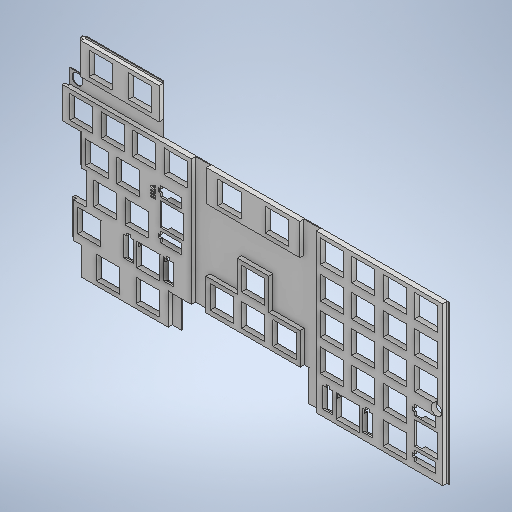
# Autodesk Inventor part: Right Plate
Saved by Autodesk Inventor 2025 (Build 290162000, 162)
## iProperties
Created: 2024-08-20
Part Number: Right Plate
Material: Generic
Document SubType Name: Modeling
Designer: adam
Density: 1 g/cm^3
Appearance: Default
Author: adam
Autodesk Inventor part; units mm, degrees
(part 1 of 2)
ref_plane "YZ Plane" through (0, 0, 0) normal (1, 0, 0) x (0, 1, 0)
ref_plane "XZ Plane" through (0, 0, 0) normal (0, 1, 0) x (-1, 0, 0)
ref_plane "XY Plane" through (0, 0, 0) normal (0, 0, 1) x (1, 0, 0)
sketch "Sketch1" plane through (0, 0, 0) normal (0, 0, 1) x (1, 0, 0)
  line L0 (490, -165) -> (40, -165) projected
  line L1 (490, -40) -> (490, -165) projected
  line L2 (40, -40) -> (490, -40) projected
  line L3 (40, -165) -> (40, -40) projected
  circle A0 centre (62.4608, -160.0704) radius 0.725 projected
  circle A1 centre (69.4608, -161.1204) radius 0.725 projected
  circle A2 centre (66.8608, -155.3704) radius 2.55 projected
  circle A3 centre (86.3368, -160.0704) radius 0.725 projected
  circle A4 centre (93.3368, -161.1204) radius 0.725 projected
  circle A5 centre (90.7368, -155.3704) radius 2.55 projected
  line L4 (118.6501, -160.3704) -> (124.6501, -160.3704) projected
  line L5 (118.6501, -145.3704) -> (118.6501, -160.3704) projected
  line L6 (124.6501, -145.3704) -> (118.6501, -145.3704) projected
  line L7 (124.6501, -160.3704) -> (124.6501, -145.3704) projected
  circle A6 centre (53.5708, -141.0204) radius 0.725 projected
  circle A7 centre (60.5708, -142.0704) radius 0.725 projected
  circle A8 centre (79.7328, -141.0204) radius 0.725 projected
  circle A9 centre (86.7328, -142.0704) radius 0.725 projected
  circle A10 centre (57.9708, -136.3204) radius 2.55 projected
  circle A11 centre (84.1328, -136.3204) radius 2.55 projected
  circle A12 centre (105.7828, -142.0704) radius 0.725 projected
  circle A13 centre (98.7828, -141.0204) radius 0.725 projected
  circle A14 centre (124.8328, -142.0704) radius 0.725 projected
  circle A15 centre (117.8328, -141.0204) radius 0.725 projected
  circle A16 centre (136.8828, -141.0204) radius 0.725 projected
  circle A17 centre (143.8828, -142.0704) radius 0.725 projected
  circle A18 centre (103.1828, -136.3204) radius 2.55 projected
  circle A19 centre (122.2328, -136.3204) radius 2.55 projected
  circle A20 centre (141.2828, -136.3204) radius 2.55 projected
  circle A21 centre (155, -160) radius 1.75 projected
  circle A22 centre (184.0001, -160.0704) radius 0.725 projected
  circle A23 centre (191.0001, -161.1204) radius 0.725 projected
  circle A24 centre (188.4001, -155.3704) radius 2.55 projected
  line L8 (252.1501, -160.3704) -> (258.1501, -160.3704) projected
  line L9 (252.1501, -145.3704) -> (252.1501, -160.3704) projected
  line L10 (258.1501, -145.3704) -> (252.1501, -145.3704) projected
  line L11 (258.1501, -160.3704) -> (258.1501, -145.3704) projected
  circle A25 centre (162.9328, -142.0704) radius 0.725 projected
  circle A26 centre (155.9328, -141.0204) radius 0.725 projected
  circle A27 centre (174.9828, -141.0204) radius 0.725 projected
  circle A28 centre (181.9828, -142.0704) radius 0.725 projected
  circle A29 centre (194.0328, -141.0204) radius 0.725 projected
  circle A30 centre (201.0328, -142.0704) radius 0.725 projected
  circle A31 centre (160.3328, -136.3204) radius 2.55 projected
  circle A32 centre (179.3828, -136.3204) radius 2.55 projected
  circle A33 centre (198.4328, -136.3204) radius 2.55 projected
  circle A34 centre (220.0828, -142.0704) radius 0.725 projected
  circle A35 centre (213.0828, -141.0204) radius 0.725 projected
  circle A36 centre (232.1368, -141.0224) radius 0.725 projected
  circle A37 centre (239.1368, -142.0724) radius 0.725 projected
  circle A38 centre (258.1768, -142.0924) radius 0.725 projected
  circle A39 centre (251.1768, -141.0424) radius 0.725 projected
  circle A40 centre (217.4828, -136.3204) radius 2.55 projected
  circle A41 centre (236.5368, -136.3224) radius 2.55 projected
  circle A42 centre (255.5768, -136.3424) radius 2.55 projected
  circle A43 centre (45, -127) radius 1.75 projected
  circle A44 centre (55.7448, -123.0204) radius 0.725 projected
  circle A45 centre (48.7448, -121.9704) radius 0.725 projected
  circle A46 centre (70.0808, -121.9704) radius 0.725 projected
  circle A47 centre (53.1448, -117.2704) radius 2.55 projected
  circle A48 centre (77.0808, -123.0204) radius 0.725 projected
  circle A49 centre (96.1308, -123.0204) radius 0.725 projected
  circle A50 centre (89.1308, -121.9704) radius 0.725 projected
  circle A51 centre (74.4808, -117.2704) radius 2.55 projected
  circle A52 centre (93.5308, -117.2704) radius 2.55 projected
  circle A53 centre (108.1808, -121.9704) radius 0.725 projected
  circle A54 centre (115.1808, -123.0204) radius 0.725 projected
  circle A55 centre (112.5808, -117.2704) radius 2.55 projected
  circle A56 centre (134.2308, -123.0204) radius 0.725 projected
  circle A57 centre (127.2308, -121.9704) radius 0.725 projected
  circle A58 centre (153.2808, -123.0204) radius 0.725 projected
  circle A59 centre (146.2808, -121.9704) radius 0.725 projected
  circle A60 centre (131.6308, -117.2704) radius 2.55 projected
  circle A61 centre (150.6808, -117.2704) radius 2.55 projected
  circle A62 centre (55.8568, -102.9204) radius 0.725 projected
  circle A63 centre (62.8568, -103.9704) radius 0.725 projected
  circle A64 centre (84.3048, -102.9204) radius 0.725 projected
  circle A65 centre (91.3048, -103.9704) radius 0.725 projected
  circle A66 centre (103.3548, -102.9204) radius 0.725 projected
  circle A67 centre (110.3548, -103.9704) radius 0.725 projected
  circle A68 centre (122.4048, -102.9204) radius 0.725 projected
  circle A69 centre (129.4048, -103.9704) radius 0.725 projected
  circle A70 centre (141.4548, -102.9204) radius 0.725 projected
  circle A71 centre (148.4548, -103.9704) radius 0.725 projected
  circle A72 centre (165.3308, -121.9704) radius 0.725 projected
  circle A73 centre (172.3308, -123.0204) radius 0.725 projected
  circle A74 centre (169.7308, -117.2704) radius 2.55 projected
  circle A75 centre (191.3808, -123.0204) radius 0.725 projected
  circle A76 centre (184.3808, -121.9704) radius 0.725 projected
  circle A77 centre (203.4308, -121.9704) radius 0.725 projected
  circle A78 centre (188.7808, -117.2704) radius 2.55 projected
  circle A79 centre (207.8308, -117.2704) radius 2.55 projected
  circle A80 centre (210.4308, -123.0204) radius 0.725 projected
  circle A81 centre (222.4808, -121.9704) radius 0.725 projected
  circle A82 centre (229.4808, -123.0204) radius 0.725 projected
  circle A83 centre (226.8808, -117.2704) radius 2.55 projected
  circle A84 centre (248.5308, -123.0204) radius 0.725 projected
  circle A85 centre (241.5308, -121.9704) radius 0.725 projected
  circle A86 centre (260.8348, -121.9704) radius 0.725 projected
  circle A87 centre (245.9308, -117.2704) radius 2.55 projected
  circle A88 centre (167.5048, -104.0492) radius 0.725 projected
  circle A89 centre (160.5048, -102.9992) radius 0.725 projected
  circle A90 centre (179.5548, -102.9204) radius 0.725 projected
  circle A91 centre (186.5548, -103.9704) radius 0.725 projected
  circle A92 centre (198.6048, -102.9204) radius 0.725 projected
  circle A93 centre (205.6048, -103.9704) radius 0.725 projected
  circle A94 centre (217.6548, -102.9204) radius 0.725 projected
  circle A95 centre (224.6548, -103.9704) radius 0.725 projected
  circle A96 centre (236.7048, -102.9204) radius 0.725 projected
  circle A97 centre (243.7048, -103.9704) radius 0.725 projected
  circle A98 centre (255.7548, -102.9204) radius 0.725 projected
  circle A99 centre (262.7548, -103.9704) radius 0.725 projected
  circle A100 centre (265, -160) radius 1.75 projected
  circle A101 centre (281.6628, -160.0704) radius 0.725 projected
  circle A102 centre (288.6628, -161.1204) radius 0.725 projected
  circle A103 centre (286.0628, -155.3704) radius 2.55 projected
  circle A104 centre (305.5388, -160.0704) radius 0.725 projected
  circle A105 centre (312.5388, -161.1204) radius 0.725 projected
  circle A106 centre (309.9388, -155.3704) radius 2.55 projected
  circle A107 centre (375, -160) radius 1.75 projected
  circle A108 centre (277.2328, -142.0704) radius 0.725 projected
  circle A109 centre (270.2328, -141.0204) radius 0.725 projected
  circle A110 centre (306.0468, -141.0204) radius 0.725 projected
  circle A111 centre (313.0468, -142.0704) radius 0.725 projected
  circle A112 centre (274.6328, -136.3204) radius 2.55 projected
  circle A113 centre (310.4468, -136.3204) radius 2.55 projected
  line L12 (295.4468, -141.3204) -> (301.4468, -141.3204) projected
  line L13 (295.4468, -126.3204) -> (295.4468, -141.3204) projected
  line L14 (301.4468, -126.3204) -> (295.4468, -126.3204) projected
  line L15 (301.4468, -141.3204) -> (301.4468, -126.3204) projected
  circle A114 centre (357.43, -142.0196) radius 0.725 projected
  circle A115 centre (350.43, -140.9696) radius 0.725 projected
  circle A116 centre (369.48, -140.9696) radius 0.725 projected
  line L16 (319.4468, -141.3204) -> (325.4468, -141.3204) projected
  line L17 (319.4468, -126.3204) -> (319.4468, -141.3204) projected
  line L18 (325.4468, -126.3204) -> (319.4468, -126.3204) projected
  line L19 (325.4468, -141.3204) -> (325.4468, -126.3204) projected
  circle A117 centre (354.83, -136.2696) radius 2.55 projected
  circle A118 centre (373.88, -136.2696) radius 2.55 projected
  circle A119 centre (426.8108, -160.0704) radius 0.725 projected
  circle A120 centre (431.2108, -155.3704) radius 2.55 projected
  line L20 (416.2108, -160.3704) -> (422.2108, -160.3704) projected
  line L21 (416.2108, -145.3704) -> (416.2108, -160.3704) projected
  line L22 (422.2108, -145.3704) -> (416.2108, -145.3704) projected
  line L23 (422.2108, -160.3704) -> (422.2108, -145.3704) projected
  circle A121 centre (433.8108, -161.1204) radius 0.725 projected
  circle A122 centre (455.2588, -160.0704) radius 0.725 projected
  circle A123 centre (462.2588, -161.1204) radius 0.725 projected
  circle A124 centre (459.6588, -155.3704) radius 2.55 projected
  line L24 (468.7088, -160.774) -> (483.7088, -160.774) projected
  line L25 (468.7088, -154.774) -> (468.7088, -160.774) projected
  line L26 (483.7088, -154.774) -> (468.7088, -154.774) projected
  line L27 (483.7088, -160.774) -> (483.7088, -154.774) projected
  line L28 (440.2108, -160.3704) -> (446.2108, -160.3704) projected
  line L29 (440.2108, -145.3704) -> (440.2108, -160.3704) projected
  line L30 (446.2108, -145.3704) -> (440.2108, -145.3704) projected
  line L31 (446.2108, -160.3704) -> (446.2108, -145.3704) projected
  circle A125 centre (483.4088, -150.174) radius 0.725 projected
  circle A126 centre (376.48, -142.0196) radius 0.725 projected
  circle A127 centre (388.53, -140.9696) radius 0.725 projected
  circle A128 centre (395.53, -142.0196) radius 0.725 projected
  circle A129 centre (417.1588, -140.922) radius 0.725 projected
  circle A130 centre (424.1588, -141.972) radius 0.725 projected
  circle A131 centre (392.93, -136.2696) radius 2.55 projected
  circle A132 centre (421.5588, -136.222) radius 2.55 projected
  circle A133 centre (443.2088, -141.972) radius 0.725 projected
  circle A134 centre (436.2088, -140.922) radius 0.725 projected
  circle A135 centre (455.2588, -140.922) radius 0.725 projected
  circle A136 centre (478.7088, -145.774) radius 2.55 projected
  circle A137 centre (462.2588, -141.972) radius 0.725 projected
  circle A138 centre (484.4588, -143.174) radius 0.725 projected
  circle A139 centre (440.6088, -136.222) radius 2.55 projected
  circle A140 centre (459.6588, -136.222) radius 2.55 projected
  line L32 (468.7088, -136.774) -> (483.7088, -136.774) projected
  line L33 (468.7088, -130.774) -> (468.7088, -136.774) projected
  line L34 (483.7088, -130.774) -> (468.7088, -130.774) projected
  line L35 (483.7088, -136.774) -> (483.7088, -130.774) projected
  circle A141 centre (267.8348, -123.0204) radius 0.725 projected
  circle A142 centre (286.8848, -123.0204) radius 0.725 projected
  circle A143 centre (279.8848, -121.9704) radius 0.725 projected
  circle A144 centre (265.2348, -117.2704) radius 2.55 projected
  circle A145 centre (284.2848, -117.2704) radius 2.55 projected
  circle A146 centre (305.9348, -123.0204) radius 0.725 projected
  circle A147 centre (298.9348, -121.9704) radius 0.725 projected
  circle A148 centre (303.3348, -117.2704) radius 2.55 projected
  line L36 (315.6708, -122.8724) -> (330.3933, -122.8724)
  line L37 (315.6708, -116.8724) -> (315.6708, -122.8724) projected
  line L38 (330.3933, -116.8724) -> (315.6708, -116.8724)
  line L39 (330.3933, -122.8724) -> (330.3933, -116.8724)
  circle A149 centre (369.48, -121.9196) radius 0.725 projected
  circle A150 centre (373.88, -117.2196) radius 2.55 projected
  circle A151 centre (274.8048, -102.9204) radius 0.725 projected
  circle A152 centre (281.8048, -103.9704) radius 0.725 projected
  circle A153 centre (293.8548, -102.9204) radius 0.725 projected
  circle A154 centre (300.8548, -103.9704) radius 0.725 projected
  circle A155 centre (329.3458, -112.2974) radius 0.725 projected
  circle A156 centre (324.6458, -107.8974) radius 2.55 projected
  circle A157 centre (330.3958, -105.2974) radius 0.725 projected
  circle A158 centre (376.48, -122.9696) radius 0.725 projected
  circle A159 centre (417.1588, -121.872) radius 0.725 projected
  circle A160 centre (424.1588, -122.922) radius 0.725 projected
  circle A161 centre (421.5588, -117.172) radius 2.55 projected
  circle A162 centre (485, -127) radius 1.75 projected
  circle A163 centre (443.2088, -122.922) radius 0.725 projected
  circle A164 centre (436.2088, -121.872) radius 0.725 projected
  circle A165 centre (455.2588, -121.872) radius 0.725 projected
  circle A166 centre (440.6088, -117.172) radius 2.55 projected
  circle A167 centre (462.2588, -122.922) radius 0.725 projected
  circle A168 centre (481.3088, -122.922) radius 0.725 projected
  circle A169 centre (474.3088, -121.872) radius 0.725 projected
  circle A170 centre (459.6588, -117.172) radius 2.55 projected
  circle A171 centre (478.7088, -117.172) radius 2.55 projected
  circle A172 centre (417.1588, -102.822) radius 0.725 projected
  circle A173 centre (424.1588, -103.872) radius 0.725 projected
  circle A174 centre (436.2088, -102.822) radius 0.725 projected
  circle A175 centre (443.2088, -103.872) radius 0.725 projected
  circle A176 centre (455.2588, -102.822) radius 0.725 projected
  circle A177 centre (462.2588, -103.872) radius 0.725 projected
  circle A178 centre (474.3088, -102.822) radius 0.725 projected
  circle A179 centre (481.3088, -103.872) radius 0.725 projected
  line L40 (45.2568, -103.2204) -> (51.2568, -103.2204) projected
  line L41 (45.2568, -88.2204) -> (45.2568, -103.2204) projected
  line L42 (51.2568, -88.2204) -> (45.2568, -88.2204) projected
  line L43 (51.2568, -103.2204) -> (51.2568, -88.2204) projected
  circle A180 centre (60.2568, -98.2204) radius 2.55 projected
  line L44 (69.2568, -103.2204) -> (75.2568, -103.2204) projected
  line L45 (69.2568, -88.2204) -> (69.2568, -103.2204) projected
  line L46 (75.2568, -88.2204) -> (69.2568, -88.2204) projected
  line L47 (75.2568, -103.2204) -> (75.2568, -88.2204) projected
  circle A181 centre (88.7048, -98.2204) radius 2.55 projected
  circle A182 centre (107.7548, -98.2204) radius 2.55 projected
  circle A183 centre (126.8048, -98.2204) radius 2.55 projected
  circle A184 centre (145.8548, -98.2204) radius 2.55 projected
  circle A185 centre (51.1288, -83.8704) radius 0.725 projected
  circle A186 centre (58.1288, -84.9204) radius 0.725 projected
  circle A187 centre (74.9068, -83.8704) radius 0.725 projected
  circle A188 centre (81.9068, -84.9204) radius 0.725 projected
  circle A189 centre (93.9568, -83.8704) radius 0.725 projected
  circle A190 centre (55.5288, -79.1704) radius 2.55 projected
  circle A191 centre (79.3068, -79.1704) radius 2.55 projected
  circle A192 centre (98.3568, -79.1704) radius 2.55 projected
  circle A193 centre (100.9568, -84.9204) radius 0.725 projected
  circle A194 centre (113.0068, -83.8704) radius 0.725 projected
  circle A195 centre (120.0068, -84.9204) radius 0.725 projected
  circle A196 centre (132.0568, -83.8704) radius 0.725 projected
  circle A197 centre (139.0568, -84.9204) radius 0.725 projected
  circle A198 centre (151.1068, -83.8704) radius 0.725 projected
  circle A199 centre (117.4068, -79.1704) radius 2.55 projected
  circle A200 centre (136.4568, -79.1704) radius 2.55 projected
  circle A201 centre (164.9048, -98.2992) radius 2.55 projected
  circle A202 centre (183.9548, -98.2204) radius 2.55 projected
  circle A203 centre (203.0048, -98.2204) radius 2.55 projected
  circle A204 centre (222.0548, -98.2204) radius 2.55 projected
  circle A205 centre (241.1048, -98.2204) radius 2.55 projected
  circle A206 centre (260.1548, -98.2204) radius 2.55 projected
  circle A207 centre (158.1068, -84.9204) radius 0.725 projected
  circle A208 centre (170.1568, -83.8704) radius 0.725 projected
  circle A209 centre (177.1568, -84.9204) radius 0.725 projected
  circle A210 centre (189.2068, -83.8704) radius 0.725 projected
  circle A211 centre (196.2068, -84.9204) radius 0.725 projected
  circle A212 centre (208.2568, -83.8704) radius 0.725 projected
  circle A213 centre (155.5068, -79.1704) radius 2.55 projected
  circle A214 centre (174.5568, -79.1704) radius 2.55 projected
  circle A215 centre (193.6068, -79.1704) radius 2.55 projected
  circle A216 centre (215.2568, -84.9204) radius 0.725 projected
  circle A217 centre (227.3068, -83.8704) radius 0.725 projected
  circle A218 centre (234.3068, -84.9204) radius 0.725 projected
  circle A219 centre (246.3568, -83.8704) radius 0.725 projected
  circle A220 centre (253.3568, -84.9204) radius 0.725 projected
  circle A221 centre (212.6568, -79.1704) radius 2.55 projected
  circle A222 centre (231.7068, -79.1704) radius 2.55 projected
  circle A223 centre (250.7568, -79.1704) radius 2.55 projected
  circle A224 centre (45, -64.8616) radius 1.75 projected
  circle A225 centre (50.8588, -50.6116) radius 2.55 projected
  circle A226 centre (81.9072, -50.3984) radius 2.55 projected
  circle A227 centre (48.2588, -44.8616) radius 0.725 projected
  circle A228 centre (55.2588, -45.9116) radius 0.725 projected
  circle A229 centre (79.3072, -44.6484) radius 0.725 projected
  circle A230 centre (86.3072, -45.6984) radius 0.725 projected
  circle A231 centre (105.7228, -50.5136) radius 2.55 projected
  circle A232 centre (129.5988, -50.5416) radius 2.55 projected
  circle A233 centre (153.4748, -50.5136) radius 2.55 projected
  circle A234 centre (103.1228, -44.7636) radius 0.725 projected
  circle A235 centre (110.1228, -45.8136) radius 0.725 projected
  circle A236 centre (126.9988, -44.7916) radius 0.725 projected
  circle A237 centre (133.9988, -45.8416) radius 0.725 projected
  circle A238 centre (150.8748, -44.7636) radius 0.725 projected
  circle A239 centre (155, -64.8616) radius 1.75 projected
  circle A240 centre (175.2648, -63.1601) radius 0.425 projected
  circle A241 centre (177.7648, -63.1601) radius 0.425 projected
  circle A242 centre (180.2648, -63.1601) radius 0.425 projected
  circle A243 centre (174.0148, -60.6601) radius 0.425 projected
  circle A244 centre (176.5148, -60.6601) radius 0.425 projected
  circle A245 centre (179.0148, -60.6601) radius 0.425 projected
  circle A246 centre (181.5148, -60.6601) radius 0.425 projected
  circle A247 centre (182.7648, -63.1601) radius 0.425 projected
  circle A248 centre (185.2648, -63.1601) radius 0.425 projected
  circle A249 centre (187.7648, -63.1601) radius 0.425 projected
  circle A250 centre (190.2648, -63.1601) radius 0.425 projected
  circle A251 centre (192.7648, -63.1601) radius 0.425 projected
  circle A252 centre (195.2648, -63.1601) radius 0.425 projected
  circle A253 centre (197.7648, -63.1601) radius 0.425 projected
  circle A254 centre (200.2648, -63.1601) radius 0.425 projected
  circle A255 centre (202.7648, -63.1601) radius 0.425 projected
  circle A256 centre (205.2648, -63.1601) radius 0.425 projected
  circle A257 centre (207.7648, -63.1601) radius 0.425 projected
  circle A258 centre (184.0148, -60.6601) radius 0.425 projected
  circle A259 centre (186.5148, -60.6601) radius 0.425 projected
  circle A260 centre (189.0148, -60.6601) radius 0.425 projected
  circle A261 centre (191.5148, -60.6601) radius 0.425 projected
  circle A262 centre (194.0148, -60.6601) radius 0.425 projected
  circle A263 centre (196.5148, -60.6601) radius 0.425 projected
  circle A264 centre (199.0148, -60.6601) radius 0.425 projected
  circle A265 centre (201.5148, -60.6601) radius 0.425 projected
  circle A266 centre (204.0148, -60.6601) radius 0.425 projected
  circle A267 centre (206.5148, -60.6601) radius 0.425 projected
  circle A268 centre (209.0148, -60.6601) radius 0.425 projected
  circle A269 centre (210.2648, -63.1601) radius 0.425 projected
  circle A270 centre (212.7648, -63.1601) radius 0.425 projected
  circle A271 centre (211.5148, -60.6601) radius 0.425 projected
  circle A272 centre (177.3508, -50.5136) radius 2.55 projected
  circle A273 centre (157.8748, -45.8136) radius 0.725 projected
  circle A274 centre (174.7508, -44.7636) radius 0.725 projected
  circle A275 centre (181.7508, -45.8136) radius 0.725 projected
  circle A276 centre (207.2568, -44.7636) radius 0.725 projected
  circle A277 centre (209.8568, -50.5136) radius 2.55 projected
  circle A278 centre (233.7388, -50.5136) radius 2.55 projected
  circle A279 centre (257.6148, -50.5136) radius 2.55 projected
  circle A280 centre (214.2568, -45.8136) radius 0.725 projected
  circle A281 centre (231.1388, -44.7636) radius 0.725 projected
  circle A282 centre (238.1388, -45.8136) radius 0.725 projected
  circle A283 centre (255.0148, -44.7636) radius 0.725 projected
  circle A284 centre (262.0148, -45.8136) radius 0.725 projected
  circle A285 centre (279.2048, -98.2204) radius 2.55 projected
  circle A286 centre (298.2548, -98.2204) radius 2.55 projected
  line L48 (315.6708, -98.8724) -> (330.6708, -98.8724) construction
  line L49 (315.6708, -92.8724) -> (315.6708, -98.8724) construction
  line L50 (330.6708, -92.8724) -> (315.6708, -92.8724) construction
  line L51 (330.6708, -98.8724) -> (330.6708, -92.8724) construction
  circle A287 centre (265.4068, -83.8704) radius 0.725 projected
  circle A288 centre (272.4068, -84.9204) radius 0.725 projected
  circle A289 centre (284.4568, -83.8704) radius 0.725 projected
  circle A290 centre (291.4568, -84.9204) radius 0.725 projected
  circle A291 centre (303.5068, -83.8704) radius 0.725 projected
  circle A292 centre (310.5068, -84.9204) radius 0.725 projected
  circle A293 centre (269.8068, -79.1704) radius 2.55 projected
  circle A294 centre (288.8568, -79.1704) radius 2.55 projected
  circle A295 centre (307.9068, -79.1704) radius 2.55 projected
  circle A296 centre (322.5568, -83.8704) radius 0.725 projected
  circle A297 centre (329.5568, -84.9204) radius 0.725 projected
  circle A298 centre (355.158, -83.8056) radius 0.725 projected
  circle A299 centre (362.158, -84.8556) radius 0.725 projected
  circle A300 centre (326.9568, -79.1704) radius 2.55 projected
  circle A301 centre (359.558, -79.1056) radius 2.55 projected
  circle A302 centre (421.5588, -98.122) radius 2.55 projected
  circle A303 centre (440.6088, -98.122) radius 2.55 projected
  circle A304 centre (459.6588, -98.122) radius 2.55 projected
  circle A305 centre (478.7088, -98.122) radius 2.55 projected
  circle A306 centre (383.754, -83.8056) radius 0.725 projected
  circle A307 centre (390.754, -84.8556) radius 0.725 projected
  circle A308 centre (417.1588, -83.772) radius 0.725 projected
  circle A309 centre (424.1588, -84.822) radius 0.725 projected
  circle A310 centre (388.154, -79.1056) radius 2.55 projected
  circle A311 centre (421.5588, -79.072) radius 2.55 projected
  circle A312 centre (436.2088, -83.772) radius 0.725 projected
  circle A313 centre (443.2088, -84.822) radius 0.725 projected
  circle A314 centre (455.2588, -83.772) radius 0.725 projected
  circle A315 centre (462.2588, -84.822) radius 0.725 projected
  circle A316 centre (474.3088, -83.772) radius 0.725 projected
  circle A317 centre (481.3088, -84.822) radius 0.725 projected
  circle A318 centre (440.6088, -79.072) radius 2.55 projected
  circle A319 centre (459.6588, -79.072) radius 2.55 projected
  circle A320 centre (478.7088, -79.072) radius 2.55 projected
  circle A321 centre (265, -64.8616) radius 1.75 projected
  circle A322 centre (375, -64.8616) radius 1.75 projected
  circle A323 centre (281.4908, -50.5136) radius 2.55 projected
  circle A324 centre (305.3668, -50.5136) radius 2.55 projected
  circle A325 centre (278.8908, -44.7636) radius 0.725 projected
  circle A326 centre (285.8908, -45.8136) radius 0.725 projected
  circle A327 centre (302.7668, -44.7636) radius 0.725 projected
  circle A328 centre (309.7668, -45.8136) radius 0.725 projected
  circle A329 centre (333.3668, -48.0136) radius 5 projected
  circle A330 centre (485, -64.8616) radius 1.75 projected
  circle A331 centre (408.3668, -48.0136) radius 5 projected
  circle A332 centre (453.2088, -50.322) radius 5 projected
  circle A333 centre (481.2088, -50.322) radius 5 projected
  circle A334 centre (432.68, -43) radius 0.5 projected
  circle A335 centre (435.22, -43) radius 0.5 projected
  circle A336 centre (437.76, -43) radius 0.5 projected
  circle A337 centre (440.3, -43) radius 0.5 projected
  line L52 (269.5528, -61.0161) -> (269.5528, -40) construction
  line L53 (260.2818, -61.0161) -> (269.5528, -61.0161) construction
  line L54 (260.2818, -88.6954) -> (260.2818, -61.0161) construction
  line L55 (269.6798, -88.6954) -> (260.2818, -88.6954) construction
  line L56 (269.6798, -107.7454) -> (269.6798, -88.6954) construction
  line L57 (274.7598, -107.7454) -> (269.6798, -107.7454) construction
  line L58 (274.7598, -126.7954) -> (274.7598, -107.7454) construction
  line L59 (265.1048, -126.7954) -> (274.7598, -126.7954) construction
  line L60 (265.1048, -148.1602) -> (265.1048, -126.7954) construction
  line L61 (272.1064, -148.1602) -> (265.1048, -148.1602) construction
  line L62 (272.1064, -165) -> (272.1064, -148.1602) construction
  line L63 (272.1064, -165) -> (272.1064, -148.1602)
  line L64 (272.1064, -148.1602) -> (265.1048, -148.1602)
  line L65 (265.1048, -148.1602) -> (265.1048, -126.7954)
  line L66 (265.1048, -126.7954) -> (274.7598, -126.7954)
  line L67 (274.7598, -126.7954) -> (274.7598, -107.7454)
  line L68 (274.7598, -107.7454) -> (269.6798, -107.7454)
  line L69 (269.6798, -107.7454) -> (269.6798, -88.6954)
  line L70 (269.6798, -88.6954) -> (260.2818, -88.6954)
  line L71 (260.2818, -88.6954) -> (260.2818, -61.0161)
  line L72 (260.2818, -61.0161) -> (269.5528, -61.0161)
  line L73 (269.5528, -61.0161) -> (269.5528, -40)
  line L74 (269.5528, -40) -> (316.8693, -40)
  line L75 (316.8693, -40) -> (316.8693, -69.6056)
  line L76 (316.8693, -69.6056) -> (490, -69.6056)
  line L77 (490, -69.6056) -> (490, -165)
  line L78 (490, -165) -> (405.2108, -165)
  line L79 (405.2108, -165) -> (405.2108, -146)
  line L80 (405.2108, -146) -> (327.9413, -146)
  line L81 (327.9413, -146) -> (327.9413, -165)
  line L82 (327.9413, -165) -> (272.1064, -165)
  line L83 (274.4883, -43.5111) -> (288.4933, -43.5111)
  line L84 (288.4933, -43.5111) -> (288.4933, -57.5161)
  line L85 (288.4933, -57.5161) -> (274.4883, -57.5161)
  line L86 (274.4883, -57.5161) -> (274.4883, -43.5111)
  line L87 (274.4883, -43.5111) -> (288.4933, -57.5161) construction
  line L88 (288.4933, -43.5111) -> (274.4883, -57.5161) construction
  line L89 (298.3643, -43.5111) -> (312.3693, -43.5111)
  line L90 (312.3693, -43.5111) -> (312.3693, -57.5161)
  line L91 (312.3693, -57.5161) -> (298.3643, -57.5161)
  line L92 (298.3643, -57.5161) -> (298.3643, -43.5111)
  line L93 (298.3643, -43.5111) -> (312.3693, -57.5161) construction
  line L94 (312.3693, -43.5111) -> (298.3643, -57.5161) construction
  line L95 (262.8043, -72.1679) -> (276.8093, -72.1679)
  line L96 (276.8093, -72.1679) -> (276.8093, -86.1729)
  line L97 (276.8093, -86.1729) -> (262.8043, -86.1729)
  line L98 (262.8043, -86.1729) -> (262.8043, -72.1679)
  line L99 (262.8043, -72.1679) -> (276.8093, -86.1729) construction
  line L100 (276.8093, -72.1679) -> (262.8043, -86.1729) construction
  line L101 (281.8543, -72.1679) -> (295.8593, -72.1679)
  line L102 (295.8593, -72.1679) -> (295.8593, -86.1729)
  line L103 (295.8593, -86.1729) -> (281.8543, -86.1729)
  line L104 (281.8543, -86.1729) -> (281.8543, -72.1679)
  line L105 (281.8543, -72.1679) -> (295.8593, -86.1729) construction
  line L106 (295.8593, -72.1679) -> (281.8543, -86.1729) construction
  line L107 (300.9043, -72.1679) -> (314.9093, -72.1679)
  line L108 (314.9093, -72.1679) -> (314.9093, -86.1729)
  line L109 (314.9093, -86.1729) -> (300.9043, -86.1729)
  line L110 (300.9043, -86.1729) -> (300.9043, -72.1679)
  line L111 (300.9043, -72.1679) -> (314.9093, -86.1729) construction
  line L112 (314.9093, -72.1679) -> (300.9043, -86.1729) construction
  line L113 (319.9543, -72.1679) -> (333.9593, -72.1679)
  line L114 (333.9593, -72.1679) -> (333.9593, -86.1729)
  line L115 (333.9593, -86.1729) -> (319.9543, -86.1729)
  line L116 (319.9543, -86.1729) -> (319.9543, -72.1679)
  line L117 (319.9543, -72.1679) -> (333.9593, -86.1729) construction
  line L118 (333.9593, -72.1679) -> (319.9543, -86.1729) construction
  line L119 (272.2023, -91.2179) -> (286.2073, -91.2179)
  line L120 (286.2073, -91.2179) -> (286.2073, -105.2229)
  line L121 (286.2073, -105.2229) -> (272.2023, -105.2229)
  line L122 (272.2023, -105.2229) -> (272.2023, -91.2179)
  line L123 (272.2023, -91.2179) -> (286.2073, -105.2229) construction
  line L124 (286.2073, -91.2179) -> (272.2023, -105.2229) construction
  line L125 (291.2523, -91.2179) -> (305.2573, -91.2179)
  line L126 (305.2573, -91.2179) -> (305.2573, -105.2229)
  line L127 (305.2573, -105.2229) -> (291.2523, -105.2229)
  line L128 (291.2523, -105.2229) -> (291.2523, -91.2179)
  line L129 (291.2523, -91.2179) -> (305.2573, -105.2229) construction
  line L130 (305.2573, -91.2179) -> (291.2523, -105.2229) construction
  line L131 (317.6433, -100.8949) -> (331.6483, -100.8949)
  line L132 (331.6483, -100.8949) -> (331.6483, -114.8999)
  line L133 (331.6483, -114.8999) -> (317.6433, -114.8999)
  line L134 (317.6433, -114.8999) -> (317.6433, -100.8949)
  line L135 (317.6433, -100.8949) -> (331.6483, -114.8999) construction
  line L136 (331.6483, -100.8949) -> (317.6433, -114.8999) construction
  line L137 (277.2823, -110.2679) -> (291.2873, -110.2679)
  line L138 (291.2873, -110.2679) -> (291.2873, -124.2729)
  line L139 (291.2873, -124.2729) -> (277.2823, -124.2729)
  line L140 (277.2823, -124.2729) -> (277.2823, -110.2679)
  line L141 (277.2823, -110.2679) -> (291.2873, -124.2729) construction
  line L142 (291.2873, -110.2679) -> (277.2823, -124.2729) construction
  line L143 (296.3323, -110.2679) -> (310.3373, -110.2679)
  line L144 (310.3373, -110.2679) -> (310.3373, -124.2729)
  line L145 (310.3373, -124.2729) -> (296.3323, -124.2729)
  line L146 (296.3323, -124.2729) -> (296.3323, -110.2679)
  line L147 (296.3323, -110.2679) -> (310.3373, -124.2729) construction
  line L148 (310.3373, -110.2679) -> (296.3323, -124.2729) construction
  line L149 (267.6303, -129.3179) -> (281.6353, -129.3179)
  line L150 (281.6353, -129.3179) -> (281.6353, -143.3229)
  line L151 (281.6353, -143.3229) -> (267.6303, -143.3229)
  line L152 (267.6303, -143.3229) -> (267.6303, -129.3179)
  line L153 (267.6303, -129.3179) -> (281.6353, -143.3229) construction
  line L154 (281.6353, -129.3179) -> (267.6303, -143.3229) construction
  line L155 (303.4443, -129.3179) -> (317.4493, -129.3179)
  line L156 (317.4493, -129.3179) -> (317.4493, -143.3229)
  line L157 (317.4493, -143.3229) -> (303.4443, -143.3229)
  line L158 (303.4443, -143.3229) -> (303.4443, -129.3179)
  line L159 (303.4443, -129.3179) -> (317.4493, -143.3229) construction
  line L160 (317.4493, -129.3179) -> (303.4443, -143.3229) construction
  line L161 (279.0603, -148.3679) -> (293.0653, -148.3679)
  line L162 (293.0653, -148.3679) -> (293.0653, -162.3729)
  line L163 (293.0653, -162.3729) -> (279.0603, -162.3729)
  line L164 (279.0603, -162.3729) -> (279.0603, -148.3679)
  line L165 (279.0603, -148.3679) -> (293.0653, -162.3729) construction
  line L166 (293.0653, -148.3679) -> (279.0603, -162.3729) construction
  line L167 (302.9363, -148.3679) -> (316.9413, -148.3679)
  line L168 (316.9413, -148.3679) -> (316.9413, -162.3729)
  line L169 (316.9413, -162.3729) -> (302.9363, -162.3729)
  line L170 (302.9363, -162.3729) -> (302.9363, -148.3679)
  line L171 (302.9363, -148.3679) -> (316.9413, -162.3729) construction
  line L172 (316.9413, -148.3679) -> (302.9363, -162.3729) construction
  line L173 (347.8275, -129.2671) -> (361.8325, -129.2671)
  line L174 (361.8325, -129.2671) -> (361.8325, -143.2721)
  line L175 (361.8325, -143.2721) -> (347.8275, -143.2721)
  line L176 (347.8275, -143.2721) -> (347.8275, -129.2671)
  line L177 (347.8275, -129.2671) -> (361.8325, -143.2721) construction
  line L178 (361.8325, -129.2671) -> (347.8275, -143.2721) construction
  line L179 (366.8775, -129.2671) -> (380.8825, -129.2671)
  line L180 (380.8825, -129.2671) -> (380.8825, -143.2721)
  line L181 (380.8825, -143.2721) -> (366.8775, -143.2721)
  line L182 (366.8775, -143.2721) -> (366.8775, -129.2671)
  line L183 (366.8775, -129.2671) -> (380.8825, -143.2721) construction
  line L184 (380.8825, -129.2671) -> (366.8775, -143.2721) construction
  line L185 (385.9275, -129.2671) -> (399.9325, -129.2671)
  line L186 (399.9325, -129.2671) -> (399.9325, -143.2721)
  line L187 (399.9325, -143.2721) -> (385.9275, -143.2721)
  line L188 (385.9275, -143.2721) -> (385.9275, -129.2671)
  line L189 (385.9275, -129.2671) -> (399.9325, -143.2721) construction
  line L190 (399.9325, -129.2671) -> (385.9275, -143.2721) construction
  line L191 (366.8775, -110.2171) -> (380.8825, -110.2171)
  line L192 (380.8825, -110.2171) -> (380.8825, -124.2221)
  line L193 (380.8825, -124.2221) -> (366.8775, -124.2221)
  line L194 (366.8775, -124.2221) -> (366.8775, -110.2171)
  line L195 (366.8775, -110.2171) -> (380.8825, -124.2221) construction
  line L196 (380.8825, -110.2171) -> (366.8775, -124.2221) construction
  line L197 (352.5555, -72.1031) -> (366.5605, -72.1031)
  line L198 (366.5605, -72.1031) -> (366.5605, -86.1081)
  line L199 (366.5605, -86.1081) -> (352.5555, -86.1081)
  line L200 (352.5555, -86.1081) -> (352.5555, -72.1031)
  line L201 (352.5555, -72.1031) -> (366.5605, -86.1081) construction
  line L202 (366.5605, -72.1031) -> (352.5555, -86.1081) construction
  line L203 (381.1515, -72.1031) -> (395.1565, -72.1031)
  line L204 (395.1565, -72.1031) -> (395.1565, -86.1081)
  line L205 (395.1565, -86.1081) -> (381.1515, -86.1081)
  line L206 (381.1515, -86.1081) -> (381.1515, -72.1031)
  line L207 (381.1515, -72.1031) -> (395.1565, -86.1081) construction
  line L208 (395.1565, -72.1031) -> (381.1515, -86.1081) construction
  line L209 (414.5563, -72.0695) -> (428.5613, -72.0695)
  line L210 (428.5613, -72.0695) -> (428.5613, -86.0745)
  line L211 (428.5613, -86.0745) -> (414.5563, -86.0745)
  line L212 (414.5563, -86.0745) -> (414.5563, -72.0695)
  line L213 (414.5563, -72.0695) -> (428.5613, -86.0745) construction
  line L214 (428.5613, -72.0695) -> (414.5563, -86.0745) construction
  line L215 (433.6063, -72.0695) -> (447.6113, -72.0695)
  line L216 (447.6113, -72.0695) -> (447.6113, -86.0745)
  line L217 (447.6113, -86.0745) -> (433.6063, -86.0745)
  line L218 (433.6063, -86.0745) -> (433.6063, -72.0695)
  line L219 (433.6063, -72.0695) -> (447.6113, -86.0745) construction
  line L220 (447.6113, -72.0695) -> (433.6063, -86.0745) construction
  line L221 (452.6563, -72.0695) -> (466.6613, -72.0695)
  line L222 (466.6613, -72.0695) -> (466.6613, -86.0745)
  line L223 (466.6613, -86.0745) -> (452.6563, -86.0745)
  line L224 (452.6563, -86.0745) -> (452.6563, -72.0695)
  line L225 (452.6563, -72.0695) -> (466.6613, -86.0745) construction
  line L226 (466.6613, -72.0695) -> (452.6563, -86.0745) construction
  line L227 (471.7063, -72.0695) -> (485.7113, -72.0695)
  line L228 (485.7113, -72.0695) -> (485.7113, -86.0745)
  line L229 (485.7113, -86.0745) -> (471.7063, -86.0745)
  line L230 (471.7063, -86.0745) -> (471.7063, -72.0695)
  line L231 (471.7063, -72.0695) -> (485.7113, -86.0745) construction
  line L232 (485.7113, -72.0695) -> (471.7063, -86.0745) construction
  line L233 (471.7063, -91.1195) -> (485.7113, -91.1195)
  line L234 (485.7113, -91.1195) -> (485.7113, -105.1245)
  line L235 (485.7113, -105.1245) -> (471.7063, -105.1245)
  line L236 (471.7063, -105.1245) -> (471.7063, -91.1195)
  line L237 (471.7063, -91.1195) -> (485.7113, -105.1245) construction
  line L238 (485.7113, -91.1195) -> (471.7063, -105.1245) construction
  line L239 (452.6563, -91.1195) -> (466.6613, -91.1195)
  line L240 (466.6613, -91.1195) -> (466.6613, -105.1245)
  line L241 (466.6613, -105.1245) -> (452.6563, -105.1245)
  line L242 (452.6563, -105.1245) -> (452.6563, -91.1195)
  line L243 (452.6563, -91.1195) -> (466.6613, -105.1245) construction
  line L244 (466.6613, -91.1195) -> (452.6563, -105.1245) construction
  line L245 (433.6063, -91.1195) -> (447.6113, -91.1195)
  line L246 (447.6113, -91.1195) -> (447.6113, -105.1245)
  line L247 (447.6113, -105.1245) -> (433.6063, -105.1245)
  line L248 (433.6063, -105.1245) -> (433.6063, -91.1195)
  line L249 (433.6063, -91.1195) -> (447.6113, -105.1245) construction
  line L250 (447.6113, -91.1195) -> (433.6063, -105.1245) construction
  line L251 (414.5563, -91.1195) -> (428.5613, -91.1195)
  line L252 (428.5613, -91.1195) -> (428.5613, -105.1245)
  line L253 (428.5613, -105.1245) -> (414.5563, -105.1245)
  line L254 (414.5563, -105.1245) -> (414.5563, -91.1195)
  line L255 (414.5563, -91.1195) -> (428.5613, -105.1245) construction
  line L256 (428.5613, -91.1195) -> (414.5563, -105.1245) construction
  line L257 (414.5563, -110.1695) -> (428.5613, -110.1695)
  line L258 (428.5613, -110.1695) -> (428.5613, -124.1745)
  line L259 (428.5613, -124.1745) -> (414.5563, -124.1745)
  line L260 (414.5563, -124.1745) -> (414.5563, -110.1695)
  line L261 (414.5563, -110.1695) -> (428.5613, -124.1745) construction
  line L262 (428.5613, -110.1695) -> (414.5563, -124.1745) construction
  line L263 (433.6063, -110.1695) -> (447.6113, -110.1695)
  line L264 (447.6113, -110.1695) -> (447.6113, -124.1745)
  line L265 (447.6113, -124.1745) -> (433.6063, -124.1745)
  line L266 (433.6063, -124.1745) -> (433.6063, -110.1695)
  line L267 (433.6063, -110.1695) -> (447.6113, -124.1745) construction
  line L268 (447.6113, -110.1695) -> (433.6063, -124.1745) construction
  line L269 (452.6563, -110.1695) -> (466.6613, -110.1695)
  line L270 (466.6613, -110.1695) -> (466.6613, -124.1745)
  line L271 (466.6613, -124.1745) -> (452.6563, -124.1745)
  line L272 (452.6563, -124.1745) -> (452.6563, -110.1695)
  line L273 (452.6563, -110.1695) -> (466.6613, -124.1745) construction
  line L274 (466.6613, -110.1695) -> (452.6563, -124.1745) construction
  line L275 (471.7063, -110.1695) -> (485.7113, -110.1695)
  line L276 (485.7113, -110.1695) -> (485.7113, -124.1745)
  line L277 (485.7113, -124.1745) -> (471.7063, -124.1745)
  line L278 (471.7063, -124.1745) -> (471.7063, -110.1695)
  line L279 (471.7063, -110.1695) -> (485.7113, -124.1745) construction
  line L280 (485.7113, -110.1695) -> (471.7063, -124.1745) construction
  line L281 (414.5563, -129.2195) -> (428.5613, -129.2195)
  line L282 (428.5613, -129.2195) -> (428.5613, -143.2245)
  line L283 (428.5613, -143.2245) -> (414.5563, -143.2245)
  line L284 (414.5563, -143.2245) -> (414.5563, -129.2195)
  line L285 (414.5563, -129.2195) -> (428.5613, -143.2245) construction
  line L286 (428.5613, -129.2195) -> (414.5563, -143.2245) construction
  line L287 (433.6063, -129.2195) -> (447.6113, -129.2195)
  line L288 (447.6113, -129.2195) -> (447.6113, -143.2245)
  line L289 (447.6113, -143.2245) -> (433.6063, -143.2245)
  line L290 (433.6063, -143.2245) -> (433.6063, -129.2195)
  line L291 (433.6063, -129.2195) -> (447.6113, -143.2245) construction
  line L292 (447.6113, -129.2195) -> (433.6063, -143.2245) construction
  line L293 (452.6563, -129.2195) -> (466.6613, -129.2195)
  line L294 (466.6613, -129.2195) -> (466.6613, -143.2245)
  line L295 (466.6613, -143.2245) -> (452.6563, -143.2245)
  line L296 (452.6563, -143.2245) -> (452.6563, -129.2195)
  line L297 (452.6563, -129.2195) -> (466.6613, -143.2245) construction
  line L298 (466.6613, -129.2195) -> (452.6563, -143.2245) construction
  line L299 (424.2083, -148.3679) -> (438.2133, -148.3679)
  line L300 (438.2133, -148.3679) -> (438.2133, -162.3729)
  line L301 (438.2133, -162.3729) -> (424.2083, -162.3729)
  line L302 (424.2083, -162.3729) -> (424.2083, -148.3679)
  line L303 (424.2083, -148.3679) -> (438.2133, -162.3729) construction
  line L304 (438.2133, -148.3679) -> (424.2083, -162.3729) construction
  line L305 (452.6563, -148.3679) -> (466.6613, -148.3679)
  line L306 (466.6613, -148.3679) -> (466.6613, -162.3729)
  line L307 (466.6613, -162.3729) -> (452.6563, -162.3729)
  line L308 (452.6563, -162.3729) -> (452.6563, -148.3679)
  line L309 (452.6563, -148.3679) -> (466.6613, -162.3729) construction
  line L310 (466.6613, -148.3679) -> (452.6563, -162.3729) construction
  line L311 (471.7063, -138.7715) -> (485.7113, -138.7715)
  line L312 (485.7113, -138.7715) -> (485.7113, -152.7765)
  line L313 (485.7113, -152.7765) -> (471.7063, -152.7765)
  line L314 (471.7063, -152.7765) -> (471.7063, -138.7715)
  line L315 (471.7063, -138.7715) -> (485.7113, -152.7765) construction
  line L316 (485.7113, -138.7715) -> (471.7063, -152.7765) construction
  circle A338 centre (485, -127) radius 3.25
  circle A339 centre (375, -160) radius 3.25
  circle A340 centre (265, -64.8616) radius 3.25
  line L317 (295.4468, -142.0679) -> (295.4468, -129.5679)
  line L318 (295.4468, -129.5679) -> (297.4468, -129.5679)
  line L319 (297.4468, -129.5679) -> (297.4468, -128.0679)
  line L320 (297.4468, -128.0679) -> (299.4468, -128.0679)
  line L321 (299.4468, -128.0679) -> (299.4468, -129.5679)
  line L322 (299.4468, -129.5679) -> (301.4468, -129.5679)
  line L323 (301.4468, -129.5679) -> (301.4468, -142.0679)
  line L324 (301.4468, -142.0679) -> (295.4468, -142.0679)
  line L325 (319.4468, -142.0679) -> (319.4468, -129.5679)
  line L326 (319.4468, -129.5679) -> (321.4468, -129.5679)
  line L327 (321.4468, -129.5679) -> (321.4468, -128.0679)
  line L328 (321.4468, -128.0679) -> (323.4468, -128.0679)
  line L329 (323.4468, -128.0679) -> (323.4468, -129.5679)
  line L330 (323.4468, -129.5679) -> (325.4468, -129.5679)
  line L331 (325.4468, -129.5679) -> (325.4468, -142.0679)
  line L332 (325.4468, -142.0679) -> (319.4468, -142.0679)
  line L333 (330.3933, -92.8724) -> (317.8933, -92.8724)
  line L334 (317.8933, -92.8724) -> (317.8933, -94.8724)
  line L335 (317.8933, -94.8724) -> (316.3933, -94.8724)
  line L336 (316.3933, -94.8724) -> (316.3933, -96.8724)
  line L337 (316.3933, -96.8724) -> (317.8933, -96.8724)
  line L338 (317.8933, -96.8724) -> (317.8933, -98.8724)
  line L339 (317.8933, -98.8724) -> (330.3933, -98.8724)
  line L340 (330.3933, -98.8724) -> (330.3933, -92.8724)
  line L341 (317.8933, -116.8724) -> (317.8933, -118.8724)
  line L342 (317.8933, -118.8724) -> (316.3933, -118.8724)
  line L343 (316.3933, -118.8724) -> (316.3933, -120.8724)
  line L344 (316.3933, -120.8724) -> (317.8933, -120.8724)
  line L345 (317.8933, -120.8724) -> (317.8933, -122.8724)
  line L346 (330.3933, -116.8724) -> (317.8933, -116.8724)
  line L347 (416.2108, -148.6179) -> (418.2108, -148.6179)
  line L348 (418.2108, -148.6179) -> (418.2108, -147.1179)
  line L349 (418.2108, -147.1179) -> (420.2108, -147.1179)
  line L350 (420.2108, -147.1179) -> (420.2108, -148.6179)
  line L351 (420.2108, -148.6179) -> (422.2108, -148.6179)
  line L352 (422.2108, -148.6179) -> (422.2108, -161.1179)
  line L353 (422.2108, -161.1179) -> (416.2108, -161.1179)
  line L354 (416.2108, -161.1179) -> (416.2108, -148.6179)
  line L355 (440.2108, -148.6179) -> (442.2108, -148.6179)
  line L356 (442.2108, -148.6179) -> (442.2108, -147.1179)
  line L357 (442.2108, -147.1179) -> (444.2108, -147.1179)
  line L358 (444.2108, -147.1179) -> (444.2108, -148.6179)
  line L359 (444.2108, -148.6179) -> (446.2108, -148.6179)
  line L360 (446.2108, -148.6179) -> (446.2108, -161.1179)
  line L361 (446.2108, -161.1179) -> (440.2108, -161.1179)
  line L362 (440.2108, -161.1179) -> (440.2108, -148.6179)
  line L363 (471.9563, -154.774) -> (471.9563, -156.774)
  line L364 (471.9563, -156.774) -> (470.4563, -156.774)
  line L365 (470.4563, -156.774) -> (470.4563, -158.774)
  line L366 (470.4563, -158.774) -> (471.9563, -158.774)
  line L367 (471.9563, -158.774) -> (471.9563, -160.774)
  line L368 (471.9563, -160.774) -> (484.4563, -160.774)
  line L369 (484.4563, -160.774) -> (484.4563, -154.774)
  line L370 (484.4563, -154.774) -> (471.9563, -154.774)
  line L371 (471.9563, -136.774) -> (471.9563, -134.774)
  line L372 (471.9563, -134.774) -> (470.4563, -134.774)
  line L373 (470.4563, -134.774) -> (470.4563, -132.774)
  line L374 (470.4563, -132.774) -> (471.9563, -132.774)
  line L375 (471.9563, -132.774) -> (471.9563, -130.774)
  line L376 (471.9563, -130.774) -> (484.4563, -130.774)
  line L377 (484.4563, -130.774) -> (484.4563, -136.774)
  line L378 (484.4563, -136.774) -> (471.9563, -136.774)
  circle A341 centre (359.558, -79.1056) radius 2.55 construction
  line L379 (330.3933, -98.8724) -> (330.3933, -116.8724) construction
  point P0 (0, 0)
  point P1 (485.7113, -123.8288)
  point P2 (483.3941, -124.1745)
  dimension "d0" = 14.005
  dimension "d1" = 14.005
  dimension "d2" = 14.005
  dimension "d3" = 14.005
  dimension "d4" = 14.005
  dimension "d5" = 14.005
  dimension "d6" = 14.005
  dimension "d7" = 14.005
  dimension "d8" = 14.005
  dimension "d9" = 14.005
  dimension "d10" = 14.005
  dimension "d11" = 14.005
  dimension "d12" = 14.005
  dimension "d13" = 14.005
  dimension "d14" = 14.005
  dimension "d15" = 14.005
  dimension "d16" = 14.005
  dimension "d17" = 14.005
  dimension "d18" = 14.005
  dimension "d19" = 14.005
  dimension "d20" = 14.005
  dimension "d21" = 14.005
  dimension "d22" = 14.005
  dimension "d23" = 14.005
  dimension "d24" = 14.005
  dimension "d25" = 14.005
  dimension "d26" = 14.005
  dimension "d27" = 14.005
  dimension "d28" = 14.005
  dimension "d29" = 14.005
  dimension "d30" = 14.005
  dimension "d31" = 14.005
  dimension "d32" = 14.005
  dimension "d33" = 14.005
  dimension "d34" = 14.005
  dimension "d35" = 14.005
  dimension "d36" = 14.005
  dimension "d37" = 14.005
  dimension "d38" = 14.005
  dimension "d39" = 14.005
  dimension "d40" = 14.005
  dimension "d41" = 14.005
  dimension "d42" = 14.005
  dimension "d43" = 14.005
  dimension "d44" = 14.005
  dimension "d45" = 14.005
  dimension "d46" = 14.005
  dimension "d47" = 14.005
  dimension "d48" = 14.005
  dimension "d49" = 14.005
  dimension "d50" = 14.005
  dimension "d51" = 14.005
  dimension "d52" = 14.005
  dimension "d53" = 14.005
  dimension "d54" = 14.005
  dimension "d55" = 14.005
  dimension "d56" = 14.005
  dimension "d57" = 14.005
  dimension "d58" = 14.005
  dimension "d59" = 14.005
  dimension "d60" = 14.005
  dimension "d61" = 14.005
  dimension "d62" = 14.005
  dimension "d63" = 14.005
  constraints: 640 end point, 86 perpendicular, 78 midpoint, 78 parallel, 42 horizontal, 39 point on line, 24 collinear, 14 equal length, 6 vertical, 3 centre point, 3 coincident, 2 equal radius
  measures "d0" distance of L84.end L85.end
  measures "d1" distance of L83.end L84.end
  measures "d2" distance of L90.end L91.end
  measures "d3" distance of L89.end L90.end
  measures "d4" distance of L96.end L97.end
  measures "d5" distance of L95.end L96.end
  measures "d6" distance of L102.end L103.end
  measures "d7" distance of L101.end L102.end
  measures "d8" distance of L108.end L109.end
  measures "d9" distance of L107.end L108.end
  measures "d10" distance of L114.end L115.end
  measures "d11" distance of L113.end L114.end
  measures "d12" distance of L120.end L121.end
  measures "d13" distance of L119.end L120.end
  measures "d14" distance of L126.end L127.end
  measures "d15" distance of L125.end L126.end
  measures "d16" distance of L132.end L133.end
  measures "d17" distance of L131.end L132.end
  measures "d18" distance of L138.end L139.end
  measures "d19" distance of L137.end L138.end
  measures "d20" distance of L144.end L145.end
  measures "d21" distance of L143.end L144.end
  measures "d22" distance of L150.end L151.end
  measures "d23" distance of L149.end L150.end
  measures "d24" distance of L156.end L157.end
  measures "d25" distance of L155.end L156.end
  measures "d26" distance of L162.end L163.end
  measures "d27" distance of L161.end L162.end
  measures "d28" distance of L168.end L169.end
  measures "d29" distance of L167.end L168.end
  measures "d30" distance of L174.end L175.end
  measures "d31" distance of L173.end L174.end
  measures "d32" distance of L180.end L181.end
  measures "d33" distance of L179.end L180.end
  measures "d34" distance of L186.end L187.end
  measures "d35" distance of L185.end L186.end
  measures "d36" distance of L192.end L193.end
  measures "d37" distance of L191.end L192.end
  measures "d38" distance of L198.end L199.end
  measures "d39" distance of L197.end L198.end
  measures "d40" distance of L204.end L205.end
  measures "d41" distance of L203.end L204.end
  measures "d42" distance of L210.end L211.end
  measures "d43" distance of L209.end L210.end
  measures "d44" distance of L216.end L217.end
  measures "d45" distance of L215.end L216.end
  measures "d46" distance of L222.end L223.end
  measures "d47" distance of L221.end L222.end
  measures "d48" distance of L228.end L229.end
  measures "d49" distance of L227.end L228.end
  measures "d50" distance of L234.end L235.end
  measures "d51" distance of L233.end L234.end
  measures "d52" distance of L240.end L241.end
  measures "d53" distance of L239.end L240.end
  measures "d54" distance of L246.end L247.end
  measures "d55" distance of L245.end L246.end
  measures "d56" distance of L252.end L253.end
  measures "d57" distance of L251.end L252.end
  measures "d58" distance of L258.end L259.end
  measures "d59" distance of L257.end L258.end
  measures "d60" distance of L264.end L265.end
  measures "d61" distance of L263.end L264.end
  measures "d62" distance of L270.end L271.end
  measures "d63" distance of L269.end L270.end
extrude "Thin base" add sketch "Sketch1" along normal blind 0.5 contours L0 L79 L80 L81 L63 L64 L65 L66 L67 L68 L69 L70 L71 L72 L73 L2 L75 L76 L1 | L13 L14 L15 L322 L321 L320 L319 L318 | L17 L18 L19 L330 L329 L328 L327 L326 | L21 L22 L23 L351 L350 L349 L348 L347 | L25 L26 L363 L364 L365 L366 L367 L24 | L29 L30 L31 L359 L358 L357 L356 L355 | L33 L34 L375 L374 L373 L372 L371 L32 | L37 L38 L341 L342 L343 L344 L345 L36 | L340 L339 L338 L337 L336 L335 L334 L333
sketch "Sketch13" plane through (0, 0, 0) normal (0, 0, -1) x (-1, 0, 0)
  line L0 (-317.6433, -114.8999) -> (-317.6433, -100.8949) construction
  line L1 (-331.6483, -100.8949) -> (-331.6483, -114.8999) construction
  line L2 (-317.6433, -107.8974) -> (-331.6483, -107.8974) construction
  line L3 (-330.3933, -116.8724) -> (-330.3933, -107.8974) construction
  line L4 (-330.3933, -107.8974) -> (-330.3933, -98.9224) construction
  line L5 (-330.3933, -98.9224) -> (-330.3933, -92.9224)
  line L6 (-330.3933, -92.9224) -> (-317.8933, -92.9224)
  line L7 (-317.8933, -92.9224) -> (-317.8933, -94.9224)
  line L8 (-317.8933, -94.9224) -> (-316.3933, -94.9224)
  line L9 (-316.3933, -94.9224) -> (-316.3933, -96.9224)
  line L10 (-316.3933, -96.9224) -> (-317.8933, -96.9224)
  line L11 (-317.8933, -96.9224) -> (-317.8933, -98.9224)
  line L12 (-317.8933, -98.9224) -> (-330.3933, -98.9224)
  line L13 (-317.8933, -118.8724) -> (-317.8933, -116.8724) construction
  line L14 (-317.8933, -116.8724) -> (-330.3933, -116.8724) construction
  line L15 (-330.3933, -116.8724) -> (-330.3933, -122.8724) construction
  line L16 (-330.3933, -122.8724) -> (-317.8933, -122.8724) construction
  line L17 (-317.8933, -122.8724) -> (-317.8933, -120.8724) construction
  line L18 (-317.8933, -120.8724) -> (-316.3933, -120.8724) construction
  line L19 (-316.3933, -120.8724) -> (-316.3933, -118.8724) construction
  line L20 (-316.3933, -118.8724) -> (-317.8933, -118.8724) construction
  point P0 (0, 0)
  constraints: 22 end point, 7 perpendicular, 6 equal length, 4 point on line, 2 midpoint, 1 vertical
extrude "Extrusion14" cut sketch "Sketch13" against normal up to surface (0.5 mm away)